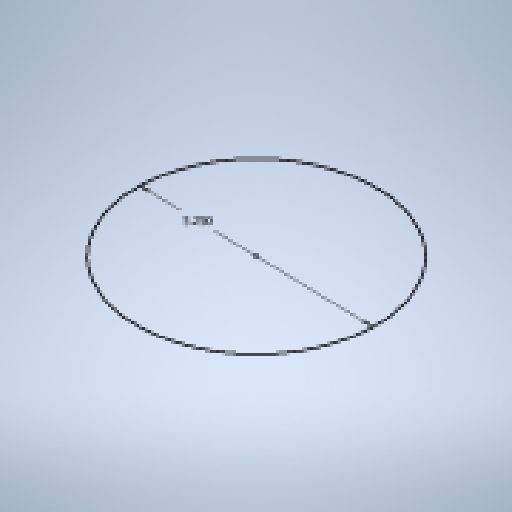
# Autodesk Inventor part: Chassis
Saved by Autodesk Inventor 2023.2 (Build 272271000, 271)
## iProperties
Created: 2023-01-05
Part Number: Chassis
Material: UHMW, White
Document SubType Name: Modeling
Designer: Nathan Cai
Mass: 112.815 g
Surface Area: 414.579 cm^2
Volume: 120.016 cm^3
Density: 0.94 g/cm^3
Appearance: Smooth - White
Author: Nathan Cai
Autodesk Inventor part; units mm, degrees
ref_plane "YZ Plane" through (0, 0, 0) normal (1, 0, 0) x (0, 1, 0)
ref_plane "XZ Plane" through (0, 0, 0) normal (0, 1, 0) x (-1, 0, 0)
ref_plane "XY Plane" through (0, 0, 0) normal (0, 0, 1) x (1, 0, 0)
sketch "Sketch1" plane through (0, 0, 0) normal (0, 1, 0) x (-1, 0, 0)
  circle A0 centre (0, 0) radius 60.325
  line L0 (0, 0) -> (0, -60.325) construction
  line L1 (58.1987, 15.875) -> (58.1987, -15.875)
  line L2 (38.1, 46.7707) -> (-38.1, 46.7707) construction
  line L3 (-38.1, 46.7707) -> (-38.1, 21.3707) construction
  line L4 (-38.1, 21.3707) -> (38.1, 21.3707)
  line L5 (38.1, 21.3707) -> (38.1, 46.7707) construction
  line L6 (38.1, 46.7707) -> (-38.1, 21.3707) construction
  line L7 (-38.1, 46.7707) -> (38.1, 21.3707) construction
  line L8 (38.1, 21.3707) -> (50.1927, 33.4634)
  circle A1 centre (42.3333, 34.0707) radius 1.7526
  line L9 (38.1, 21.3707) -> (44.5387, 40.6867) construction
  line L10 (38.1, 34.0707) -> (42.3333, 34.0707) construction
  line L11 (-38.1, 21.3707) -> (-50.1927, 33.4634)
  circle A2 centre (-42.3333, 34.0707) radius 1.7526
  line L12 (34.925, -30.1369) -> (-34.925, -30.1369)
  line L13 (-34.925, -30.1369) -> (-34.925, -49.1869) construction
  line L14 (-34.925, -49.1869) -> (34.925, -49.1869) construction
  line L15 (34.925, -49.1869) -> (34.925, -30.1369) construction
  line L16 (34.925, -30.1369) -> (-34.925, -49.1869) construction
  line L17 (-34.925, -30.1369) -> (34.925, -49.1869) construction
  line L18 (34.925, -30.1369) -> (40.8344, -44.4034)
  circle A3 centre (34.925, -39.6619) radius 1.7526
  line L19 (-34.925, -30.1369) -> (-40.8344, -44.4034)
  circle A4 centre (-34.925, -39.6619) radius 1.7526
  line L20 (-58.1987, 15.875) -> (-58.1987, -15.875)
  circle A5 centre (0, 0) radius 69.85
  line L21 (48.3346, 36.0954) -> (36.7849, 24.5457)
  line L22 (36.7849, 24.5457) -> (-36.7849, 24.5457)
  line L23 (-36.7849, 24.5457) -> (-48.3346, 36.0954)
  arc A6 (40.0883, 36.3157) -> (43.279, 31.0398) centre (42.3333, 34.0707) ccw
  line L24 (44.5008, 40.7282) -> (40.0883, 36.3157)
  arc A7 (-43.279, 31.0398) -> (-40.0883, 36.3157) centre (-42.3333, 34.0707) ccw
  line L25 (-44.5008, 40.7282) -> (-40.0883, 36.3157)
  line L26 (-38.3079, -46.6006) -> (-32.8035, -33.3119)
  line L27 (-32.8035, -33.3119) -> (32.8035, -33.3119)
  line L28 (32.8035, -33.3119) -> (38.3079, -46.6006)
  circle A8 centre (-34.925, -39.6619) radius 3.175
  circle A9 centre (34.925, -39.6619) radius 3.175
  point P0 (0, 34.0707)
  point P1 (0, -39.6619)
  point P2 (-36.5609, -42.383)
  point P3 (-34.1576, -36.581)
  point P4 (34.1576, -36.581)
  point P5 (36.5609, -42.383)
  dimension "d0" = 120.65
  dimension "d1" = 31.75
  dimension "d2" = 76.2
  dimension "d3" = 25.4
  dimension "d4" = 45
  dimension "d5" = 3.5052
  dimension "d7" = 69.85
  dimension "d8" = 19.05
  dimension "d9" = 22.5
  dimension "d10" = 3.5052
  dimension "d11" = 9.525
  dimension "d12" = 3.175
  dimension "d13" = 3.175
  dimension "d14" = 3.175
  dimension "d15" = 6.35
  dimension "d16" = 3.175
  dimension "d17" = 3.175
  dimension "d18" = 3.175
  dimension "d19" = 6.35
  dimension "d20" = 6.35
  constraints: 58 end point, 10 symmetric about line, 9 centre point, 6 midpoint, 5 parallel, 4 coincident, 4 point on circle, 3 horizontal, 3 perpendicular, 3 point on line, 2 vertical, 1 tangent, 19 other
  measures "d1" distance of L1.start L1.end
  measures "d2" distance of L4.end L3.end
  measures "d3" distance of L3.end L2.end
  measures "d4" angle of L5 L8
  measures "d5" diameter of A1
  measures "d7" distance of L14.end L13.end
  measures "d8" distance of L13.end L12.end
  measures "d9" angle of L15 L18
  measures "d10" diameter of A3
  measures "d12" distance between parallel lines of L8 L21
  measures "d13" distance between parallel lines of L4 L22
  measures "d14" distance between parallel lines of L11 L23
  measures "d15" diameter of A6
  measures "d16" distance between parallel lines of L12 L27
  measures "d17" distance between parallel lines of L18 L28
  measures "d18" distance between parallel lines of L19 L26
  measures "d19" diameter of A8
  measures "d20" diameter of A9
extrude "Extrusion1" add sketch "Sketch1" along normal blind 25.4 contours A0 L1 | L8 L4 L11 A0 L23 L22 L21 | A0 L28 A9 L27 L26 A8 L19 L12 L18 | L21 A6 L24 A0 | A9 L28 A3 | L28 A3 A9 | L25 A7 L23 A0 | A8 L26 A4 | L26 A4 A8 | L20 A0 | A5
fillet "Fillet1" radius 3.175 22 edges at (-43.279, 12.7, 31.0398) (-44.5008, 12.7, 40.7282) (-36.7849, 12.7, 24.5457) (36.7849, 12.7, 24.5457) (43.279, 12.7, 31.0398) (44.5008, 12.7, 40.7282) (-38.3079, 12.7, -46.6006) (-36.5609, 12.7, -42.383) (-34.1576, 12.7, -36.581) (-32.8035, 12.7, -33.3119) (38.3079, 12.7, -46.6006) (36.5609, 12.7, -42.383) (34.1576, 12.7, -36.581) (32.8035, 12.7, -33.3119) (40.8344, 12.7, -44.4034) (-40.8344, 12.7, -44.4034) (-50.1927, 12.7, 33.4634) (50.1927, 12.7, 33.4634) (34.925, 12.7, -30.1369) (-34.925, 12.7, -30.1369) (-38.1, 12.7, 21.3707) (38.1, 12.7, 21.3707)
fillet "Fillet2" radius 12.7 4 edges at (58.1987, 12.7, 15.875) (58.1987, 12.7, -15.875) (-58.1987, 12.7, 15.875) (-58.1987, 12.7, -15.875)
sketch "Sketch2" plane through (-58.1987, 0, 14.0715) normal (1, 0, 0) x (0, 0, -1)
  line L0 (14.0715, 0) -> (14.0715, 25.4) construction
  line L1 (0, 25.4) -> (28.1431, 25.4) projected
  circle A0 centre (14.0715, 12.7) radius 4.7625
  dimension "d25" = 9.525
  constraints: 2 end point, 2 midpoint, 1 centre point
  measures "d25" diameter of A0
extrude "Extrusion2" cut sketch "Sketch2" along normal through all both and the other way through all
equation "\"d9\" = 0.5 * d4"
equation "\"d13\" = d12"
equation "\"d14\" = d13"
equation "\"d17\" = d16"
equation "\"d18\" = d16"
body "Solid1"
